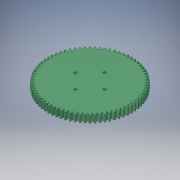
# Autodesk Inventor part: 000.302 - Втулка
Saved by Autodesk Inventor 2019 (Build 230136000, 136)
## iProperties
Created: 2020-02-27
Part Number: 000.302 - Втулка
Material: Пластик АБС
Document SubType Name: Modeling
Designer: Петров Иван
Density: 1.06 g/cm^3
Appearance: Гладкий — темный цвет морской волны
Author: Петров Иван
Autodesk Inventor part; units mm, degrees
ref_plane "YZ Plane" through (0, 0, 0) normal (1, 0, 0) x (0, 1, 0)
ref_plane "XZ Plane" through (0, 0, 0) normal (0, 1, 0) x (-1, 0, 0)
ref_plane "XY Plane" through (0, 0, 0) normal (0, 0, 1) x (1, 0, 0)
sketch "Эскиз1" plane through (0, 0, 0) normal (0, 1, 0) x (-1, 0, 0)
  circle A0 centre (0, 0) radius 12.5
  dimension "d0" = 25
  constraints: 1 centre point, 1 coincident
  measures "d0" diameter of A0
extrude "Выдавливание1" add sketch "Эскиз1" along normal blind 8
sketch "Эскиз2" plane through (0, 8, 0) normal (0, 1, 0) x (1, 0, 0)
  circle A0 centre (0, 0) radius 23
  dimension "d3" = 46
  constraints: 1 centre point, 1 coincident
  measures "d3" diameter of A0
extrude "Выдавливание2" add sketch "Эскиз2" along normal blind 2
sketch "Эскиз3" plane through (0, 10, 0) normal (0, 1, 0) x (1, 0, 0)
  arc A0 (-8.1938, 41.193) -> (-8.7829, 35.8928) centre (15.46, 35.881) ccw
  arc A1 (-8.7829, 35.8928) -> (-10.3402, 35.4755) centre (0, 0) ccw
  arc A2 (-10.3402, 35.4755) -> (-13.5005, 39.7711) centre (-31.3293, 23.3439) ccw
  arc A3 (-13.5005, 39.7711) -> (-15.2224, 39.1443) centre (0, 0) ccw
  arc A4 (-15.2224, 39.1443) -> (-14.8822, 33.8224) centre (8.9945, 38.0205) ccw
  arc A5 (-14.8822, 33.8224) -> (-16.3433, 33.141) centre (0, 0) ccw
  arc A6 (-16.3433, 33.141) -> (-20.2015, 36.8225) centre (-34.9069, 17.549) ccw
  arc A7 (-20.2015, 36.8225) -> (-21.7885, 35.9063) centre (0, 0) ccw
  arc A8 (-21.7885, 35.9063) -> (-20.5293, 30.7243) centre (2.2556, 39.0048) ccw
  arc A9 (-20.5293, 30.7243) -> (-21.8499, 29.7995) centre (0, 0) ccw
  arc A10 (-21.8499, 29.7995) -> (-26.2888, 32.7551) centre (-37.424, 11.2208) ccw
  arc A11 (-26.2888, 32.7551) -> (-27.6925, 31.5773) centre (0, 0) ccw
  arc A12 (-27.6925, 31.5773) -> (-25.5526, 26.6926) centre (-4.5518, 38.8039) ccw
  arc A13 (-25.5526, 26.6926) -> (-26.6926, 25.5526) centre (0, 0) ccw
  arc A14 (-26.6926, 25.5526) -> (-31.5773, 27.6925) centre (-38.8039, 4.5518) ccw
  arc A15 (-31.5773, 27.6925) -> (-32.7551, 26.2888) centre (0, 0) ccw
  arc A16 (-32.7551, 26.2888) -> (-29.7995, 21.8499) centre (-11.2208, 37.424) ccw
  arc A17 (-29.7995, 21.8499) -> (-30.7243, 20.5293) centre (0, 0) ccw
  arc A18 (-30.7243, 20.5293) -> (-35.9063, 21.7885) centre (-39.0048, -2.2556) ccw
  arc A19 (-35.9063, 21.7885) -> (-36.8225, 20.2015) centre (0, 0) ccw
  arc A20 (-36.8225, 20.2015) -> (-33.141, 16.3433) centre (-17.549, 34.9069) ccw
  arc A21 (-33.141, 16.3433) -> (-33.8224, 14.8822) centre (0, 0) ccw
  arc A22 (-33.8224, 14.8822) -> (-39.1443, 15.2224) centre (-38.0205, -8.9945) ccw
  arc A23 (-39.1443, 15.2224) -> (-39.7711, 13.5005) centre (0, 0) ccw
  arc A24 (-39.7711, 13.5005) -> (-35.4755, 10.3402) centre (-23.3439, 31.3293) ccw
  arc A25 (-35.4755, 10.3402) -> (-35.8928, 8.7829) centre (0, 0) ccw
  arc A26 (-35.8928, 8.7829) -> (-41.193, 8.1938) centre (-35.881, -15.46) ccw
  arc A27 (-41.193, 8.1938) -> (-41.5112, 6.3892) centre (0, 0) ccw
  arc A28 (-41.5112, 6.3892) -> (-36.7321, 4.0228) centre (-28.4295, 26.7997) ccw
  arc A29 (-36.7321, 4.0228) -> (-36.8726, 2.4168) centre (0, 0) ccw
  arc A30 (-36.8726, 2.4168) -> (-41.99, 0.9162) centre (-32.6513, -21.4558) ccw
  arc A31 (-41.99, 0.9162) -> (-41.99, -0.9162) centre (0, 0) ccw
  arc A32 (-41.99, -0.9162) -> (-36.8726, -2.4168) centre (-32.6513, 21.4558) ccw
  arc A33 (-36.8726, -2.4168) -> (-36.7321, -4.0228) centre (0, 0) ccw
  arc A34 (-36.7321, -4.0228) -> (-41.5112, -6.3892) centre (-28.4295, -26.7997) ccw
  arc A35 (-41.5112, -6.3892) -> (-41.193, -8.1938) centre (0, 0) ccw
  arc A36 (-41.193, -8.1938) -> (-35.8928, -8.7829) centre (-35.881, 15.46) ccw
  arc A37 (-35.8928, -8.7829) -> (-35.4755, -10.3402) centre (0, 0) ccw
  arc A38 (-35.4755, -10.3402) -> (-39.7711, -13.5005) centre (-23.3439, -31.3293) ccw
  arc A39 (-39.7711, -13.5005) -> (-39.1443, -15.2224) centre (0, 0) ccw
  arc A40 (-39.1443, -15.2224) -> (-33.8224, -14.8822) centre (-38.0205, 8.9945) ccw
  arc A41 (-33.8224, -14.8822) -> (-33.141, -16.3433) centre (0, 0) ccw
  arc A42 (-33.141, -16.3433) -> (-36.8225, -20.2015) centre (-17.549, -34.9069) ccw
  arc A43 (-36.8225, -20.2015) -> (-35.9063, -21.7885) centre (0, 0) ccw
  arc A44 (-35.9063, -21.7885) -> (-30.7243, -20.5293) centre (-39.0048, 2.2556) ccw
  arc A45 (-30.7243, -20.5293) -> (-29.7995, -21.8499) centre (0, 0) ccw
  arc A46 (-29.7995, -21.8499) -> (-32.7551, -26.2888) centre (-11.2208, -37.424) ccw
  arc A47 (-32.7551, -26.2888) -> (-31.5773, -27.6925) centre (0, 0) ccw
  arc A48 (-31.5773, -27.6925) -> (-26.6926, -25.5526) centre (-38.8039, -4.5518) ccw
  arc A49 (-26.6926, -25.5526) -> (-25.5526, -26.6926) centre (0, 0) ccw
  arc A50 (-25.5526, -26.6926) -> (-27.6925, -31.5773) centre (-4.5518, -38.8039) ccw
  arc A51 (-27.6925, -31.5773) -> (-26.2888, -32.7551) centre (0, 0) ccw
  arc A52 (-26.2888, -32.7551) -> (-21.8499, -29.7995) centre (-37.424, -11.2208) ccw
  arc A53 (-21.8499, -29.7995) -> (-20.5293, -30.7243) centre (0, 0) ccw
  arc A54 (-20.5293, -30.7243) -> (-21.7885, -35.9063) centre (2.2556, -39.0048) ccw
  arc A55 (-21.7885, -35.9063) -> (-20.2015, -36.8225) centre (0, 0) ccw
  arc A56 (-20.2015, -36.8225) -> (-16.3433, -33.141) centre (-34.9069, -17.549) ccw
  arc A57 (-16.3433, -33.141) -> (-14.8822, -33.8224) centre (0, 0) ccw
  arc A58 (-14.8822, -33.8224) -> (-15.2224, -39.1443) centre (8.9945, -38.0205) ccw
  arc A59 (-15.2224, -39.1443) -> (-13.5005, -39.7711) centre (0, 0) ccw
  arc A60 (-13.5005, -39.7711) -> (-10.3402, -35.4755) centre (-31.3293, -23.3439) ccw
  arc A61 (-10.3402, -35.4755) -> (-8.7829, -35.8928) centre (0, 0) ccw
  arc A62 (-8.7829, -35.8928) -> (-8.1938, -41.193) centre (15.46, -35.881) ccw
  arc A63 (-8.1938, -41.193) -> (-6.3892, -41.5112) centre (0, 0) ccw
  arc A64 (-6.3892, -41.5112) -> (-4.0228, -36.7321) centre (-26.7997, -28.4295) ccw
  arc A65 (-4.0228, -36.7321) -> (-2.4168, -36.8726) centre (0, 0) ccw
  arc A66 (-2.4168, -36.8726) -> (-0.9162, -41.99) centre (21.4558, -32.6513) ccw
  arc A67 (-0.9162, -41.99) -> (0.9162, -41.99) centre (0, 0) ccw
  arc A68 (0.9162, -41.99) -> (2.4168, -36.8726) centre (-21.4558, -32.6513) ccw
  arc A69 (2.4168, -36.8726) -> (4.0228, -36.7321) centre (0, 0) ccw
  arc A70 (4.0228, -36.7321) -> (6.3892, -41.5112) centre (26.7997, -28.4295) ccw
  arc A71 (6.3892, -41.5112) -> (8.1938, -41.193) centre (0, 0) ccw
  arc A72 (8.1938, -41.193) -> (8.7829, -35.8928) centre (-15.46, -35.881) ccw
  arc A73 (8.7829, -35.8928) -> (10.3402, -35.4755) centre (0, 0) ccw
  arc A74 (10.3402, -35.4755) -> (13.5005, -39.7711) centre (31.3293, -23.3439) ccw
  arc A75 (13.5005, -39.7711) -> (15.2224, -39.1443) centre (0, 0) ccw
  arc A76 (15.2224, -39.1443) -> (14.8822, -33.8224) centre (-8.9945, -38.0205) ccw
  arc A77 (14.8822, -33.8224) -> (16.3433, -33.141) centre (0, 0) ccw
  arc A78 (16.3433, -33.141) -> (20.2015, -36.8225) centre (34.9069, -17.549) ccw
  arc A79 (20.2015, -36.8225) -> (21.7885, -35.9063) centre (0, 0) ccw
  arc A80 (21.7885, -35.9063) -> (20.5293, -30.7243) centre (-2.2556, -39.0048) ccw
  arc A81 (20.5293, -30.7243) -> (21.8499, -29.7995) centre (0, 0) ccw
  arc A82 (21.8499, -29.7995) -> (26.2888, -32.7551) centre (37.424, -11.2208) ccw
  arc A83 (26.2888, -32.7551) -> (27.6925, -31.5773) centre (0, 0) ccw
  arc A84 (27.6925, -31.5773) -> (25.5526, -26.6926) centre (4.5518, -38.8039) ccw
  arc A85 (25.5526, -26.6926) -> (26.6926, -25.5526) centre (0, 0) ccw
  arc A86 (26.6926, -25.5526) -> (31.5773, -27.6925) centre (38.8039, -4.5518) ccw
  arc A87 (31.5773, -27.6925) -> (32.7551, -26.2888) centre (0, 0) ccw
  arc A88 (32.7551, -26.2888) -> (29.7995, -21.8499) centre (11.2208, -37.424) ccw
  arc A89 (29.7995, -21.8499) -> (30.7243, -20.5293) centre (0, 0) ccw
  arc A90 (30.7243, -20.5293) -> (35.9063, -21.7885) centre (39.0048, 2.2556) ccw
  arc A91 (35.9063, -21.7885) -> (36.8225, -20.2015) centre (0, 0) ccw
  arc A92 (36.8225, -20.2015) -> (33.141, -16.3433) centre (17.549, -34.9069) ccw
  arc A93 (33.141, -16.3433) -> (33.8224, -14.8822) centre (0, 0) ccw
  arc A94 (33.8224, -14.8822) -> (39.1443, -15.2224) centre (38.0205, 8.9945) ccw
  arc A95 (39.1443, -15.2224) -> (39.7711, -13.5005) centre (0, 0) ccw
  arc A96 (39.7711, -13.5005) -> (35.4755, -10.3402) centre (23.3439, -31.3293) ccw
  arc A97 (35.4755, -10.3402) -> (35.8928, -8.7829) centre (0, 0) ccw
  arc A98 (35.8928, -8.7829) -> (41.193, -8.1938) centre (35.881, 15.46) ccw
  arc A99 (41.193, -8.1938) -> (41.5112, -6.3892) centre (0, 0) ccw
  arc A100 (41.5112, -6.3892) -> (36.7321, -4.0228) centre (28.4295, -26.7997) ccw
  arc A101 (36.7321, -4.0228) -> (36.8726, -2.4168) centre (0, 0) ccw
  arc A102 (36.8726, -2.4168) -> (41.99, -0.9162) centre (32.6513, 21.4558) ccw
  arc A103 (41.99, -0.9162) -> (41.99, 0.9162) centre (0, 0) ccw
  arc A104 (41.99, 0.9162) -> (36.8726, 2.4168) centre (32.6513, -21.4558) ccw
  arc A105 (36.8726, 2.4168) -> (36.7321, 4.0228) centre (0, 0) ccw
  arc A106 (36.7321, 4.0228) -> (41.5112, 6.3892) centre (28.4295, 26.7997) ccw
  arc A107 (41.5112, 6.3892) -> (41.193, 8.1938) centre (0, 0) ccw
  arc A108 (41.193, 8.1938) -> (35.8928, 8.7829) centre (35.881, -15.46) ccw
  arc A109 (35.8928, 8.7829) -> (35.4755, 10.3402) centre (0, 0) ccw
  arc A110 (35.4755, 10.3402) -> (39.7711, 13.5005) centre (23.3439, 31.3293) ccw
  arc A111 (39.7711, 13.5005) -> (39.1443, 15.2224) centre (0, 0) ccw
  arc A112 (39.1443, 15.2224) -> (33.8224, 14.8822) centre (38.0205, -8.9945) ccw
  arc A113 (33.8224, 14.8822) -> (33.141, 16.3433) centre (0, 0) ccw
  arc A114 (33.141, 16.3433) -> (36.8225, 20.2015) centre (17.549, 34.9069) ccw
  arc A115 (36.8225, 20.2015) -> (35.9063, 21.7885) centre (0, 0) ccw
  arc A116 (35.9063, 21.7885) -> (30.7243, 20.5293) centre (39.0048, -2.2556) ccw
  arc A117 (30.7243, 20.5293) -> (29.7995, 21.8499) centre (0, 0) ccw
  arc A118 (29.7995, 21.8499) -> (32.7551, 26.2888) centre (11.2208, 37.424) ccw
  arc A119 (32.7551, 26.2888) -> (31.5773, 27.6925) centre (0, 0) ccw
  arc A120 (31.5773, 27.6925) -> (26.6926, 25.5526) centre (38.8039, 4.5518) ccw
  arc A121 (26.6926, 25.5526) -> (25.5526, 26.6926) centre (0, 0) ccw
  arc A122 (25.5526, 26.6926) -> (27.6925, 31.5773) centre (4.5518, 38.8039) ccw
  arc A123 (27.6925, 31.5773) -> (26.2888, 32.7551) centre (0, 0) ccw
  arc A124 (26.2888, 32.7551) -> (21.8499, 29.7995) centre (37.424, 11.2208) ccw
  arc A125 (21.8499, 29.7995) -> (20.5293, 30.7243) centre (0, 0) ccw
  arc A126 (20.5293, 30.7243) -> (21.7885, 35.9063) centre (-2.2556, 39.0048) ccw
  arc A127 (21.7885, 35.9063) -> (20.2015, 36.8225) centre (0, 0) ccw
  arc A128 (20.2015, 36.8225) -> (16.3433, 33.141) centre (34.9069, 17.549) ccw
  arc A129 (16.3433, 33.141) -> (14.8822, 33.8224) centre (0, 0) ccw
  arc A130 (14.8822, 33.8224) -> (15.2224, 39.1443) centre (-8.9945, 38.0205) ccw
  arc A131 (15.2224, 39.1443) -> (13.5005, 39.7711) centre (0, 0) ccw
  arc A132 (13.5005, 39.7711) -> (10.3402, 35.4755) centre (31.3293, 23.3439) ccw
  arc A133 (10.3402, 35.4755) -> (8.7829, 35.8928) centre (0, 0) ccw
  arc A134 (8.7829, 35.8928) -> (8.1938, 41.193) centre (-15.46, 35.881) ccw
  arc A135 (8.1938, 41.193) -> (6.3892, 41.5112) centre (0, 0) ccw
  arc A136 (6.3892, 41.5112) -> (4.0228, 36.7321) centre (26.7997, 28.4295) ccw
  arc A137 (4.0228, 36.7321) -> (2.4168, 36.8726) centre (0, 0) ccw
  arc A138 (2.4168, 36.8726) -> (0.9162, 41.99) centre (-21.4558, 32.6513) ccw
  arc A139 (0.9162, 41.99) -> (-0.9162, 41.99) centre (0, 0) ccw
  arc A140 (-0.9162, 41.99) -> (-2.4168, 36.8726) centre (21.4558, 32.6513) ccw
  arc A141 (-2.4168, 36.8726) -> (-4.0228, 36.7321) centre (0, 0) ccw
  arc A142 (-4.0228, 36.7321) -> (-6.3892, 41.5112) centre (-26.7997, 28.4295) ccw
  arc A143 (-6.3892, 41.5112) -> (-8.1938, 41.193) centre (0, 0) ccw
  arc A144 (4.8028, -48.7641) -> (5.506, -45.6664) centre (-12.0114, -43.3185) ccw
  arc A145 (5.506, -45.6664) -> (6.5009, -45.5354) centre (0, 0) ccw
  arc A146 (6.5009, -45.5354) -> (7.9819, -48.3455) centre (22.8137, -38.7337) ccw
  arc A147 (7.9819, -48.3455) -> (9.0346, -48.1599) centre (0, 0) ccw
  arc A148 (9.0346, -48.1599) -> (9.4652, -45.0127) centre (-8.1902, -44.2005) ccw
  arc A149 (9.4652, -45.0127) -> (10.4449, -44.7955) centre (0, 0) ccw
  arc A150 (10.4449, -44.7955) -> (12.1651, -47.4659) centre (26.1028, -36.598) ccw
  arc A151 (12.1651, -47.4659) -> (13.1977, -47.1892) centre (0, 0) ccw
  arc A152 (13.1977, -47.1892) -> (13.3523, -44.0165) centre (-4.3067, -44.7461) ccw
  arc A153 (13.3523, -44.0165) -> (14.3093, -43.7148) centre (0, 0) ccw
  arc A154 (14.3093, -43.7148) -> (16.2557, -46.225) centre (29.1932, -34.1837) ccw
  arc A155 (16.2557, -46.225) -> (17.2603, -45.8594) centre (0, 0) ccw
  arc A156 (17.2603, -45.8594) -> (17.1377, -42.6853) centre (-0.3904, -44.9512) ccw
  arc A157 (17.1377, -42.6853) -> (18.0648, -42.3013) centre (0, 0) ccw
  arc A158 (18.0648, -42.3013) -> (20.2226, -44.6323) centre (32.0614, -31.5092) ccw
  arc A159 (20.2226, -44.6323) -> (21.1915, -44.1806) centre (0, 0) ccw
  arc A160 (21.1915, -44.1806) -> (20.7928, -41.0292) centre (3.5288, -44.8142) ccw
  arc A161 (20.7928, -41.0292) -> (21.6829, -40.5658) centre (0, 0) ccw
  arc A162 (21.6829, -40.5658) -> (24.0357, -42.7) centre (34.6856, -28.595) ccw
  arc A163 (24.0357, -42.7) -> (24.9614, -42.1655) centre (0, 0) ccw
  arc A164 (24.9614, -42.1655) -> (24.2896, -39.0609) centre (7.4212, -44.3361) ccw
  arc A165 (24.2896, -39.0609) -> (25.1359, -38.5217) centre (0, 0) ccw
  arc A166 (25.1359, -38.5217) -> (27.6657, -40.4426) centre (37.0458, -25.4632) ccw
  arc A167 (27.6657, -40.4426) -> (28.5414, -39.8295) centre (0, 0) ccw
  arc A168 (28.5414, -39.8295) -> (27.6016, -36.7952) centre (11.2571, -43.5206) ccw
  arc A169 (27.6016, -36.7952) -> (28.3977, -36.1844) centre (0, 0) ccw
  arc A170 (28.3977, -36.1844) -> (31.0853, -37.8775) centre (39.1241, -22.1375) ccw
  arc A171 (31.0853, -37.8775) -> (31.9042, -37.1904) centre (0, 0) ccw
  arc A172 (31.9042, -37.1904) -> (30.7034, -34.2496) centre (15.0073, -42.3739) ccw
  arc A173 (30.7034, -34.2496) -> (31.4433, -33.5717) centre (0, 0) ccw
  arc A174 (31.4433, -33.5717) -> (34.2682, -35.0241) centre (40.9046, -18.6434) ccw
  arc A175 (34.2682, -35.0241) -> (35.0241, -34.2682) centre (0, 0) ccw
  arc A176 (35.0241, -34.2682) -> (33.5717, -31.4433) centre (18.6434, -40.9046) ccw
  arc A177 (33.5717, -31.4433) -> (34.2496, -30.7034) centre (0, 0) ccw
  arc A178 (34.2496, -30.7034) -> (37.1904, -31.9042) centre (42.3739, -15.0073) ccw
  arc A179 (37.1904, -31.9042) -> (37.8775, -31.0853) centre (0, 0) ccw
  arc A180 (37.8775, -31.0853) -> (36.1844, -28.3977) centre (22.1375, -39.1241) ccw
  arc A181 (36.1844, -28.3977) -> (36.7952, -27.6016) centre (0, 0) ccw
  arc A182 (36.7952, -27.6016) -> (39.8295, -28.5414) centre (43.5206, -11.2571) ccw
  arc A183 (39.8295, -28.5414) -> (40.4426, -27.6657) centre (0, 0) ccw
  arc A184 (40.4426, -27.6657) -> (38.5217, -25.1359) centre (25.4632, -37.0458) ccw
  arc A185 (38.5217, -25.1359) -> (39.0609, -24.2896) centre (0, 0) ccw
  arc A186 (39.0609, -24.2896) -> (42.1655, -24.9614) centre (44.3361, -7.4212) ccw
  arc A187 (42.1655, -24.9614) -> (42.7, -24.0357) centre (0, 0) ccw
  arc A188 (42.7, -24.0357) -> (40.5658, -21.6829) centre (28.595, -34.6856) ccw
  arc A189 (40.5658, -21.6829) -> (41.0292, -20.7928) centre (0, 0) ccw
  arc A190 (41.0292, -20.7928) -> (44.1806, -21.1915) centre (44.8142, -3.5288) ccw
  arc A191 (44.1806, -21.1915) -> (44.6323, -20.2226) centre (0, 0) ccw
  arc A192 (44.6323, -20.2226) -> (42.3013, -18.0648) centre (31.5092, -32.0614) ccw
  arc A193 (42.3013, -18.0648) -> (42.6853, -17.1377) centre (0, 0) ccw
  arc A194 (42.6853, -17.1377) -> (45.8594, -17.2603) centre (44.9512, 0.3904) ccw
  arc A195 (45.8594, -17.2603) -> (46.225, -16.2557) centre (0, 0) ccw
  arc A196 (46.225, -16.2557) -> (43.7148, -14.3093) centre (34.1837, -29.1932) ccw
  arc A197 (43.7148, -14.3093) -> (44.0165, -13.3523) centre (0, 0) ccw
  arc A198 (44.0165, -13.3523) -> (47.1892, -13.1977) centre (44.7461, 4.3067) ccw
  arc A199 (47.1892, -13.1977) -> (47.4659, -12.1651) centre (0, 0) ccw
  arc A200 (47.4659, -12.1651) -> (44.7955, -10.4449) centre (36.598, -26.1028) ccw
  arc A201 (44.7955, -10.4449) -> (45.0127, -9.4652) centre (0, 0) ccw
  arc A202 (45.0127, -9.4652) -> (48.1599, -9.0346) centre (44.2005, 8.1902) ccw
  arc A203 (48.1599, -9.0346) -> (48.3455, -7.9819) centre (0, 0) ccw
  arc A204 (48.3455, -7.9819) -> (45.5354, -6.5009) centre (38.7337, -22.8137) ccw
  arc A205 (45.5354, -6.5009) -> (45.6664, -5.506) centre (0, 0) ccw
  arc A206 (45.6664, -5.506) -> (48.7641, -4.8028) centre (43.3185, 12.0114) ccw
  arc A207 (48.7641, -4.8028) -> (48.8572, -3.7379) centre (0, 0) ccw
  arc A208 (48.8572, -3.7379) -> (45.9287, -2.5075) centre (40.5746, -19.3511) ccw
  arc A209 (45.9287, -2.5075) -> (45.9725, -1.505) centre (0, 0) ccw
  arc A210 (45.9725, -1.505) -> (48.9971, -0.5345) centre (42.1068, 15.7411) ccw
  arc A211 (48.9971, -0.5345) -> (48.9971, 0.5345) centre (0, 0) ccw
  arc A212 (48.9971, 0.5345) -> (45.9725, 1.505) centre (42.1068, -15.7411) ccw
  arc A213 (45.9725, 1.505) -> (45.9287, 2.5075) centre (0, 0) ccw
  arc A214 (45.9287, 2.5075) -> (48.8572, 3.7379) centre (40.5746, 19.3511) ccw
  arc A215 (48.8572, 3.7379) -> (48.7641, 4.8028) centre (0, 0) ccw
  arc A216 (48.7641, 4.8028) -> (45.6664, 5.506) centre (43.3185, -12.0114) ccw
  arc A217 (45.6664, 5.506) -> (45.5354, 6.5009) centre (0, 0) ccw
  arc A218 (45.5354, 6.5009) -> (48.3455, 7.9819) centre (38.7337, 22.8137) ccw
  arc A219 (48.3455, 7.9819) -> (48.1599, 9.0346) centre (0, 0) ccw
  arc A220 (48.1599, 9.0346) -> (45.0127, 9.4652) centre (44.2005, -8.1902) ccw
  arc A221 (45.0127, 9.4652) -> (44.7955, 10.4449) centre (0, 0) ccw
  arc A222 (44.7955, 10.4449) -> (47.4659, 12.1651) centre (36.598, 26.1028) ccw
  arc A223 (47.4659, 12.1651) -> (47.1892, 13.1977) centre (0, 0) ccw
  arc A224 (47.1892, 13.1977) -> (44.0165, 13.3523) centre (44.7461, -4.3067) ccw
  arc A225 (44.0165, 13.3523) -> (43.7148, 14.3093) centre (0, 0) ccw
  arc A226 (43.7148, 14.3093) -> (46.225, 16.2557) centre (34.1837, 29.1932) ccw
  arc A227 (46.225, 16.2557) -> (45.8594, 17.2603) centre (0, 0) ccw
  arc A228 (45.8594, 17.2603) -> (42.6853, 17.1377) centre (44.9512, -0.3904) ccw
  arc A229 (42.6853, 17.1377) -> (42.3013, 18.0648) centre (0, 0) ccw
  arc A230 (42.3013, 18.0648) -> (44.6323, 20.2226) centre (31.5092, 32.0614) ccw
  arc A231 (44.6323, 20.2226) -> (44.1806, 21.1915) centre (0, 0) ccw
  arc A232 (44.1806, 21.1915) -> (41.0292, 20.7928) centre (44.8142, 3.5288) ccw
  arc A233 (41.0292, 20.7928) -> (40.5658, 21.6829) centre (0, 0) ccw
  arc A234 (40.5658, 21.6829) -> (42.7, 24.0357) centre (28.595, 34.6856) ccw
  arc A235 (42.7, 24.0357) -> (42.1655, 24.9614) centre (0, 0) ccw
  arc A236 (42.1655, 24.9614) -> (39.0609, 24.2896) centre (44.3361, 7.4212) ccw
  arc A237 (39.0609, 24.2896) -> (38.5217, 25.1359) centre (0, 0) ccw
  arc A238 (38.5217, 25.1359) -> (40.4426, 27.6657) centre (25.4632, 37.0458) ccw
  arc A239 (40.4426, 27.6657) -> (39.8295, 28.5414) centre (0, 0) ccw
  arc A240 (39.8295, 28.5414) -> (36.7952, 27.6016) centre (43.5206, 11.2571) ccw
  arc A241 (36.7952, 27.6016) -> (36.1844, 28.3977) centre (0, 0) ccw
  arc A242 (36.1844, 28.3977) -> (37.8775, 31.0853) centre (22.1375, 39.1241) ccw
  arc A243 (37.8775, 31.0853) -> (37.1904, 31.9042) centre (0, 0) ccw
  arc A244 (37.1904, 31.9042) -> (34.2496, 30.7034) centre (42.3739, 15.0073) ccw
  arc A245 (34.2496, 30.7034) -> (33.5717, 31.4433) centre (0, 0) ccw
  arc A246 (33.5717, 31.4433) -> (35.0241, 34.2682) centre (18.6434, 40.9046) ccw
  arc A247 (35.0241, 34.2682) -> (34.2682, 35.0241) centre (0, 0) ccw
  arc A248 (34.2682, 35.0241) -> (31.4433, 33.5717) centre (40.9046, 18.6434) ccw
  arc A249 (31.4433, 33.5717) -> (30.7034, 34.2496) centre (0, 0) ccw
  arc A250 (30.7034, 34.2496) -> (31.9042, 37.1904) centre (15.0073, 42.3739) ccw
  arc A251 (31.9042, 37.1904) -> (31.0853, 37.8775) centre (0, 0) ccw
  arc A252 (31.0853, 37.8775) -> (28.3977, 36.1844) centre (39.1241, 22.1375) ccw
  arc A253 (28.3977, 36.1844) -> (27.6016, 36.7952) centre (0, 0) ccw
  arc A254 (27.6016, 36.7952) -> (28.5414, 39.8295) centre (11.2571, 43.5206) ccw
  arc A255 (28.5414, 39.8295) -> (27.6657, 40.4426) centre (0, 0) ccw
  arc A256 (27.6657, 40.4426) -> (25.1359, 38.5217) centre (37.0458, 25.4632) ccw
  arc A257 (25.1359, 38.5217) -> (24.2896, 39.0609) centre (0, 0) ccw
  arc A258 (24.2896, 39.0609) -> (24.9614, 42.1655) centre (7.4212, 44.3361) ccw
  arc A259 (24.9614, 42.1655) -> (24.0357, 42.7) centre (0, 0) ccw
  arc A260 (24.0357, 42.7) -> (21.6829, 40.5658) centre (34.6856, 28.595) ccw
  arc A261 (21.6829, 40.5658) -> (20.7928, 41.0292) centre (0, 0) ccw
  arc A262 (20.7928, 41.0292) -> (21.1915, 44.1806) centre (3.5288, 44.8142) ccw
  arc A263 (21.1915, 44.1806) -> (20.2226, 44.6323) centre (0, 0) ccw
  arc A264 (20.2226, 44.6323) -> (18.0648, 42.3013) centre (32.0614, 31.5092) ccw
  arc A265 (18.0648, 42.3013) -> (17.1377, 42.6853) centre (0, 0) ccw
  arc A266 (17.1377, 42.6853) -> (17.2603, 45.8594) centre (-0.3904, 44.9512) ccw
  arc A267 (17.2603, 45.8594) -> (16.2557, 46.225) centre (0, 0) ccw
  arc A268 (16.2557, 46.225) -> (14.3093, 43.7148) centre (29.1932, 34.1837) ccw
  arc A269 (14.3093, 43.7148) -> (13.3523, 44.0165) centre (0, 0) ccw
  arc A270 (13.3523, 44.0165) -> (13.1977, 47.1892) centre (-4.3067, 44.7461) ccw
  arc A271 (13.1977, 47.1892) -> (12.1651, 47.4659) centre (0, 0) ccw
  arc A272 (12.1651, 47.4659) -> (10.4449, 44.7955) centre (26.1028, 36.598) ccw
  arc A273 (10.4449, 44.7955) -> (9.4652, 45.0127) centre (0, 0) ccw
  arc A274 (9.4652, 45.0127) -> (9.0346, 48.1599) centre (-8.1902, 44.2005) ccw
  arc A275 (9.0346, 48.1599) -> (7.9819, 48.3455) centre (0, 0) ccw
  arc A276 (7.9819, 48.3455) -> (6.5009, 45.5354) centre (22.8137, 38.7337) ccw
  arc A277 (6.5009, 45.5354) -> (5.506, 45.6664) centre (0, 0) ccw
  arc A278 (5.506, 45.6664) -> (4.8028, 48.7641) centre (-12.0114, 43.3185) ccw
  arc A279 (4.8028, 48.7641) -> (3.7379, 48.8572) centre (0, 0) ccw
  arc A280 (3.7379, 48.8572) -> (2.5075, 45.9287) centre (19.3511, 40.5746) ccw
  arc A281 (2.5075, 45.9287) -> (1.505, 45.9725) centre (0, 0) ccw
  arc A282 (1.505, 45.9725) -> (0.5345, 48.9971) centre (-15.7411, 42.1068) ccw
  arc A283 (0.5345, 48.9971) -> (-0.5345, 48.9971) centre (0, 0) ccw
  arc A284 (-0.5345, 48.9971) -> (-1.505, 45.9725) centre (15.7411, 42.1068) ccw
  arc A285 (-1.505, 45.9725) -> (-2.5075, 45.9287) centre (0, 0) ccw
  arc A286 (-2.5075, 45.9287) -> (-3.7379, 48.8572) centre (-19.3511, 40.5746) ccw
  arc A287 (3.7379, -48.8572) -> (4.8028, -48.7641) centre (0, 0) ccw
  arc A288 (-4.8028, 48.7641) -> (-5.506, 45.6664) centre (12.0114, 43.3185) ccw
  arc A289 (-5.506, 45.6664) -> (-6.5009, 45.5354) centre (0, 0) ccw
  arc A290 (-6.5009, 45.5354) -> (-7.9819, 48.3455) centre (-22.8137, 38.7337) ccw
  arc A291 (-7.9819, 48.3455) -> (-9.0346, 48.1599) centre (0, 0) ccw
  arc A292 (-9.0346, 48.1599) -> (-9.4652, 45.0127) centre (8.1902, 44.2005) ccw
  arc A293 (-9.4652, 45.0127) -> (-10.4449, 44.7955) centre (0, 0) ccw
  arc A294 (-10.4449, 44.7955) -> (-12.1651, 47.4659) centre (-26.1028, 36.598) ccw
  arc A295 (-12.1651, 47.4659) -> (-13.1977, 47.1892) centre (0, 0) ccw
  arc A296 (-13.1977, 47.1892) -> (-13.3523, 44.0165) centre (4.3067, 44.7461) ccw
  arc A297 (-13.3523, 44.0165) -> (-14.3093, 43.7148) centre (0, 0) ccw
  arc A298 (-14.3093, 43.7148) -> (-16.2557, 46.225) centre (-29.1932, 34.1837) ccw
  arc A299 (-16.2557, 46.225) -> (-17.2603, 45.8594) centre (0, 0) ccw
  arc A300 (-17.2603, 45.8594) -> (-17.1377, 42.6853) centre (0.3904, 44.9512) ccw
  arc A301 (-17.1377, 42.6853) -> (-18.0648, 42.3013) centre (0, 0) ccw
  arc A302 (-18.0648, 42.3013) -> (-20.2226, 44.6323) centre (-32.0614, 31.5092) ccw
  arc A303 (-20.2226, 44.6323) -> (-21.1915, 44.1806) centre (0, 0) ccw
  arc A304 (-21.1915, 44.1806) -> (-20.7928, 41.0292) centre (-3.5288, 44.8142) ccw
  arc A305 (-20.7928, 41.0292) -> (-21.6829, 40.5658) centre (0, 0) ccw
  arc A306 (-21.6829, 40.5658) -> (-24.0357, 42.7) centre (-34.6856, 28.595) ccw
  arc A307 (-24.0357, 42.7) -> (-24.9614, 42.1655) centre (0, 0) ccw
  arc A308 (-24.9614, 42.1655) -> (-24.2896, 39.0609) centre (-7.4212, 44.3361) ccw
  arc A309 (-24.2896, 39.0609) -> (-25.1359, 38.5217) centre (0, 0) ccw
  arc A310 (-25.1359, 38.5217) -> (-27.6657, 40.4426) centre (-37.0458, 25.4632) ccw
  arc A311 (-27.6657, 40.4426) -> (-28.5414, 39.8295) centre (0, 0) ccw
  arc A312 (-28.5414, 39.8295) -> (-27.6016, 36.7952) centre (-11.2571, 43.5206) ccw
  arc A313 (-27.6016, 36.7952) -> (-28.3977, 36.1844) centre (0, 0) ccw
  arc A314 (-28.3977, 36.1844) -> (-31.0853, 37.8775) centre (-39.1241, 22.1375) ccw
  arc A315 (-31.0853, 37.8775) -> (-31.9042, 37.1904) centre (0, 0) ccw
  arc A316 (-31.9042, 37.1904) -> (-30.7034, 34.2496) centre (-15.0073, 42.3739) ccw
  arc A317 (-30.7034, 34.2496) -> (-31.4433, 33.5717) centre (0, 0) ccw
  arc A318 (-31.4433, 33.5717) -> (-34.2682, 35.0241) centre (-40.9046, 18.6434) ccw
  arc A319 (-34.2682, 35.0241) -> (-35.0241, 34.2682) centre (0, 0) ccw
  arc A320 (-35.0241, 34.2682) -> (-33.5717, 31.4433) centre (-18.6434, 40.9046) ccw
  arc A321 (-33.5717, 31.4433) -> (-34.2496, 30.7034) centre (0, 0) ccw
  arc A322 (-34.2496, 30.7034) -> (-37.1904, 31.9042) centre (-42.3739, 15.0073) ccw
  arc A323 (-37.1904, 31.9042) -> (-37.8775, 31.0853) centre (0, 0) ccw
  arc A324 (-37.8775, 31.0853) -> (-36.1844, 28.3977) centre (-22.1375, 39.1241) ccw
  arc A325 (-36.1844, 28.3977) -> (-36.7952, 27.6016) centre (0, 0) ccw
  arc A326 (-36.7952, 27.6016) -> (-39.8295, 28.5414) centre (-43.5206, 11.2571) ccw
  arc A327 (-39.8295, 28.5414) -> (-40.4426, 27.6657) centre (0, 0) ccw
  arc A328 (-40.4426, 27.6657) -> (-38.5217, 25.1359) centre (-25.4632, 37.0458) ccw
  arc A329 (-38.5217, 25.1359) -> (-39.0609, 24.2896) centre (0, 0) ccw
  arc A330 (-39.0609, 24.2896) -> (-42.1655, 24.9614) centre (-44.3361, 7.4212) ccw
  arc A331 (-42.1655, 24.9614) -> (-42.7, 24.0357) centre (0, 0) ccw
  arc A332 (-42.7, 24.0357) -> (-40.5658, 21.6829) centre (-28.595, 34.6856) ccw
  arc A333 (-40.5658, 21.6829) -> (-41.0292, 20.7928) centre (0, 0) ccw
  arc A334 (-41.0292, 20.7928) -> (-44.1806, 21.1915) centre (-44.8142, 3.5288) ccw
  arc A335 (-44.1806, 21.1915) -> (-44.6323, 20.2226) centre (0, 0) ccw
  arc A336 (-44.6323, 20.2226) -> (-42.3013, 18.0648) centre (-31.5092, 32.0614) ccw
  arc A337 (-42.3013, 18.0648) -> (-42.6853, 17.1377) centre (0, 0) ccw
  arc A338 (-42.6853, 17.1377) -> (-45.8594, 17.2603) centre (-44.9512, -0.3904) ccw
  arc A339 (-45.8594, 17.2603) -> (-46.225, 16.2557) centre (0, 0) ccw
  arc A340 (-46.225, 16.2557) -> (-43.7148, 14.3093) centre (-34.1837, 29.1932) ccw
  arc A341 (-43.7148, 14.3093) -> (-44.0165, 13.3523) centre (0, 0) ccw
  arc A342 (-44.0165, 13.3523) -> (-47.1892, 13.1977) centre (-44.7461, -4.3067) ccw
  arc A343 (-47.1892, 13.1977) -> (-47.4659, 12.1651) centre (0, 0) ccw
  arc A344 (-47.4659, 12.1651) -> (-44.7955, 10.4449) centre (-36.598, 26.1028) ccw
  arc A345 (-44.7955, 10.4449) -> (-45.0127, 9.4652) centre (0, 0) ccw
  arc A346 (-45.0127, 9.4652) -> (-48.1599, 9.0346) centre (-44.2005, -8.1902) ccw
  arc A347 (-48.1599, 9.0346) -> (-48.3455, 7.9819) centre (0, 0) ccw
  arc A348 (-48.3455, 7.9819) -> (-45.5354, 6.5009) centre (-38.7337, 22.8137) ccw
  arc A349 (-45.5354, 6.5009) -> (-45.6664, 5.506) centre (0, 0) ccw
  arc A350 (-45.6664, 5.506) -> (-48.7641, 4.8028) centre (-43.3185, -12.0114) ccw
  arc A351 (-48.7641, 4.8028) -> (-48.8572, 3.7379) centre (0, 0) ccw
  arc A352 (-48.8572, 3.7379) -> (-45.9287, 2.5075) centre (-40.5746, 19.3511) ccw
  arc A353 (-45.9287, 2.5075) -> (-45.9725, 1.505) centre (0, 0) ccw
  arc A354 (-45.9725, 1.505) -> (-48.9971, 0.5345) centre (-42.1068, -15.7411) ccw
  arc A355 (-48.9971, 0.5345) -> (-48.9971, -0.5345) centre (0, 0) ccw
  arc A356 (-48.9971, -0.5345) -> (-45.9725, -1.505) centre (-42.1068, 15.7411) ccw
  arc A357 (-45.9725, -1.505) -> (-45.9287, -2.5075) centre (0, 0) ccw
  arc A358 (-45.9287, -2.5075) -> (-48.8572, -3.7379) centre (-40.5746, -19.3511) ccw
  arc A359 (-48.8572, -3.7379) -> (-48.7641, -4.8028) centre (0, 0) ccw
  arc A360 (-48.7641, -4.8028) -> (-45.6664, -5.506) centre (-43.3185, 12.0114) ccw
  arc A361 (-45.6664, -5.506) -> (-45.5354, -6.5009) centre (0, 0) ccw
  arc A362 (-45.5354, -6.5009) -> (-48.3455, -7.9819) centre (-38.7337, -22.8137) ccw
  arc A363 (-48.3455, -7.9819) -> (-48.1599, -9.0346) centre (0, 0) ccw
  arc A364 (-48.1599, -9.0346) -> (-45.0127, -9.4652) centre (-44.2005, 8.1902) ccw
  arc A365 (-45.0127, -9.4652) -> (-44.7955, -10.4449) centre (0, 0) ccw
  arc A366 (-44.7955, -10.4449) -> (-47.4659, -12.1651) centre (-36.598, -26.1028) ccw
  arc A367 (-47.4659, -12.1651) -> (-47.1892, -13.1977) centre (0, 0) ccw
  arc A368 (-47.1892, -13.1977) -> (-44.0165, -13.3523) centre (-44.7461, 4.3067) ccw
  arc A369 (-44.0165, -13.3523) -> (-43.7148, -14.3093) centre (0, 0) ccw
  arc A370 (-43.7148, -14.3093) -> (-46.225, -16.2557) centre (-34.1837, -29.1932) ccw
  arc A371 (-46.225, -16.2557) -> (-45.8594, -17.2603) centre (0, 0) ccw
  arc A372 (-45.8594, -17.2603) -> (-42.6853, -17.1377) centre (-44.9512, 0.3904) ccw
  arc A373 (-42.6853, -17.1377) -> (-42.3013, -18.0648) centre (0, 0) ccw
  arc A374 (-42.3013, -18.0648) -> (-44.6323, -20.2226) centre (-31.5092, -32.0614) ccw
  arc A375 (-44.6323, -20.2226) -> (-44.1806, -21.1915) centre (0, 0) ccw
  arc A376 (-44.1806, -21.1915) -> (-41.0292, -20.7928) centre (-44.8142, -3.5288) ccw
  arc A377 (-41.0292, -20.7928) -> (-40.5658, -21.6829) centre (0, 0) ccw
  arc A378 (-40.5658, -21.6829) -> (-42.7, -24.0357) centre (-28.595, -34.6856) ccw
  arc A379 (-42.7, -24.0357) -> (-42.1655, -24.9614) centre (0, 0) ccw
  arc A380 (-42.1655, -24.9614) -> (-39.0609, -24.2896) centre (-44.3361, -7.4212) ccw
  arc A381 (-39.0609, -24.2896) -> (-38.5217, -25.1359) centre (0, 0) ccw
  arc A382 (-38.5217, -25.1359) -> (-40.4426, -27.6657) centre (-25.4632, -37.0458) ccw
  arc A383 (-40.4426, -27.6657) -> (-39.8295, -28.5414) centre (0, 0) ccw
  arc A384 (-39.8295, -28.5414) -> (-36.7952, -27.6016) centre (-43.5206, -11.2571) ccw
  arc A385 (-36.7952, -27.6016) -> (-36.1844, -28.3977) centre (0, 0) ccw
  arc A386 (-36.1844, -28.3977) -> (-37.8775, -31.0853) centre (-22.1375, -39.1241) ccw
  arc A387 (-37.8775, -31.0853) -> (-37.1904, -31.9042) centre (0, 0) ccw
  arc A388 (-37.1904, -31.9042) -> (-34.2496, -30.7034) centre (-42.3739, -15.0073) ccw
  arc A389 (-34.2496, -30.7034) -> (-33.5717, -31.4433) centre (0, 0) ccw
  arc A390 (-33.5717, -31.4433) -> (-35.0241, -34.2682) centre (-18.6434, -40.9046) ccw
  arc A391 (-35.0241, -34.2682) -> (-34.2682, -35.0241) centre (0, 0) ccw
  arc A392 (-34.2682, -35.0241) -> (-31.4433, -33.5717) centre (-40.9046, -18.6434) ccw
  arc A393 (-31.4433, -33.5717) -> (-30.7034, -34.2496) centre (0, 0) ccw
  arc A394 (-30.7034, -34.2496) -> (-31.9042, -37.1904) centre (-15.0073, -42.3739) ccw
  arc A395 (-31.9042, -37.1904) -> (-31.0853, -37.8775) centre (0, 0) ccw
  arc A396 (-31.0853, -37.8775) -> (-28.3977, -36.1844) centre (-39.1241, -22.1375) ccw
  arc A397 (-28.3977, -36.1844) -> (-27.6016, -36.7952) centre (0, 0) ccw
  arc A398 (-27.6016, -36.7952) -> (-28.5414, -39.8295) centre (-11.2571, -43.5206) ccw
  arc A399 (-28.5414, -39.8295) -> (-27.6657, -40.4426) centre (0, 0) ccw
  arc A400 (-27.6657, -40.4426) -> (-25.1359, -38.5217) centre (-37.0458, -25.4632) ccw
  arc A401 (-25.1359, -38.5217) -> (-24.2896, -39.0609) centre (0, 0) ccw
  arc A402 (-24.2896, -39.0609) -> (-24.9614, -42.1655) centre (-7.4212, -44.3361) ccw
  arc A403 (-24.9614, -42.1655) -> (-24.0357, -42.7) centre (0, 0) ccw
  arc A404 (-24.0357, -42.7) -> (-21.6829, -40.5658) centre (-34.6856, -28.595) ccw
  arc A405 (-21.6829, -40.5658) -> (-20.7928, -41.0292) centre (0, 0) ccw
  arc A406 (-20.7928, -41.0292) -> (-21.1915, -44.1806) centre (-3.5288, -44.8142) ccw
  arc A407 (-21.1915, -44.1806) -> (-20.2226, -44.6323) centre (0, 0) ccw
  arc A408 (-20.2226, -44.6323) -> (-18.0648, -42.3013) centre (-32.0614, -31.5092) ccw
  arc A409 (-18.0648, -42.3013) -> (-17.1377, -42.6853) centre (0, 0) ccw
  arc A410 (-17.1377, -42.6853) -> (-17.2603, -45.8594) centre (0.3904, -44.9512) ccw
  arc A411 (-17.2603, -45.8594) -> (-16.2557, -46.225) centre (0, 0) ccw
  arc A412 (-16.2557, -46.225) -> (-14.3093, -43.7148) centre (-29.1932, -34.1837) ccw
  arc A413 (-14.3093, -43.7148) -> (-13.3523, -44.0165) centre (0, 0) ccw
  arc A414 (-13.3523, -44.0165) -> (-13.1977, -47.1892) centre (4.3067, -44.7461) ccw
  arc A415 (-13.1977, -47.1892) -> (-12.1651, -47.4659) centre (0, 0) ccw
  arc A416 (-12.1651, -47.4659) -> (-10.4449, -44.7955) centre (-26.1028, -36.598) ccw
  arc A417 (-10.4449, -44.7955) -> (-9.4652, -45.0127) centre (0, 0) ccw
  arc A418 (-9.4652, -45.0127) -> (-9.0346, -48.1599) centre (8.1902, -44.2005) ccw
  arc A419 (-9.0346, -48.1599) -> (-7.9819, -48.3455) centre (0, 0) ccw
  arc A420 (-7.9819, -48.3455) -> (-6.5009, -45.5354) centre (-22.8137, -38.7337) ccw
  arc A421 (-6.5009, -45.5354) -> (-5.506, -45.6664) centre (0, 0) ccw
  arc A422 (-5.506, -45.6664) -> (-4.8028, -48.7641) centre (12.0114, -43.3185) ccw
  arc A423 (-4.8028, -48.7641) -> (-3.7379, -48.8572) centre (0, 0) ccw
  arc A424 (-3.7379, -48.8572) -> (-2.5075, -45.9287) centre (-19.3511, -40.5746) ccw
  arc A425 (-2.5075, -45.9287) -> (-1.505, -45.9725) centre (0, 0) ccw
  arc A426 (-1.505, -45.9725) -> (-0.5345, -48.9971) centre (15.7411, -42.1068) ccw
  arc A427 (-0.5345, -48.9971) -> (0.5345, -48.9971) centre (0, 0) ccw
  arc A428 (0.5345, -48.9971) -> (1.505, -45.9725) centre (-15.7411, -42.1068) ccw
  arc A429 (1.505, -45.9725) -> (2.5075, -45.9287) centre (0, 0) ccw
  arc A430 (2.5075, -45.9287) -> (3.7379, -48.8572) centre (19.3511, -40.5746) ccw
  arc A431 (-3.7379, 48.8572) -> (-4.8028, 48.7641) centre (0, 0) ccw
  constraints: 864 point on circle, 432 centre point
extrude "Выдавливание3" add sketch "Эскиз3" along normal blind 8 contours A143 A142 A141 A140 A139 A138 A137 A136 A135 A134 A133 A132 A131 A130 A129 A128 A127 A126 A125 A124 A123 A122 A121 A120 A119 A118 A117 A116 A115 A114 A113 A112 A111 A110 A109 A108 A107 A106 A105 A104 A103 A102 A101 A100 A99 A98 A97 A96 A95 A94 A93 A92 A91 A90 A89 A88 A87 A86 A85 A84 A83 A82 A81 A80 A79 A78 A77 A76 A75 A74 A73 A72 A71 A70 A69 A68 A67 A66 A65 A64 A63 A62 A61 A60 A59 A58 A57 A56 A55 A54 A53 A52 A51 A50 A49 A48 A47 A46 A45 A44 A43 A42 A41 A40 A39 A38 A37 A36 A35 A34 A33 A32 A31 A30 A29 A28 A27 A26 A25 A24 A23 A22 A21 A20 A19 A18 A17 A16 A15 A14 A13 A12 A11 A10 A9 A8 A7 A6 A5 A4 A3 A2 A1 A0 | A287 A430 A429 A428 A427 A426 A425 A424 A423 A422 A421 A420 A419 A418 A417 A416 A415 A414 A413 A412 A411 A410 A409 A408 A407 A406 A405 A404 A403 A402 A401 A400 A399 A398 A397 A396 A395 A394 A393 A392 A391 A390 A389 A388 A387 A386 A385 A384 A383 A382 A381 A380 A379 A378 A377 A376 A375 A374 A373 A372 A371 A370 A369 A368 A367 A366 A365 A364 A363 A362 A361 A360 A359 A358 A357 A356 A355 A354 A353 A352 A351 A350 A349 A348 A347 A346 A345 A344 A343 A342 A341 A340 A339 A338 A337 A336 A335 A334 A333 A332 A331 A330 A329 A328 A327 A326 A325 A324 A323 A322 A321 A320 A319 A318 A317 A316 A315 A314 A313 A312 A311 A310 A309 A308 A307 A306 A305 A304 A303 A302 A301 A300 A299 A298 A297 A296 A295 A294 A293 A292 A291 A290 A289 A288 A431 A286 A285 A284 A283 A282 A281 A280 A279 A278 A277 A276 A275 A274 A273 A272 A271 A270 A269 A268 A267 A266 A265 A264 A263 A262 A261 A260 A259 A258 A257 A256 A255 A254 A253 A252 A251 A250 A249 A248 A247 A246 A245 A244 A243 A242 A241 A240 A239 A238 A237 A236 A235 A234 A233 A232 A231 A230 A229 A228 A227 A226 A225 A224 A223 A222 A221 A220 A219 A218 A217 A216 A215 A214 A213 A212 A211 A210 A209 A208 A207 A206 A205 A204 A203 A202 A201 A200 A199 A198 A197 A196 A195 A194 A193 A192 A191 A190 A189 A188 A187 A186 A185 A184 A183 A182 A181 A180 A179 A178 A177 A176 A175 A174 A173 A172 A171 A170 A169 A168 A167 A166 A165 A164 A163 A162 A161 A160 A159 A158 A157 A156 A155 A154 A153 A152 A151 A150 A149 A148 A147 A146 A145 A144
sketch "Эскиз4" plane through (0, 8, 0) normal (0, -1, 0) x (1, 0, 0)
  line L0 (0, 0) -> (0, -17)
  line L1 (4, -17) -> (2, -20.4641)
  line L2 (2, -20.4641) -> (-2, -20.4641)
  line L3 (-2, -20.4641) -> (-4, -17)
  line L4 (-4, -17) -> (-2, -13.5359)
  line L5 (-2, -13.5359) -> (2, -13.5359)
  line L6 (2, -13.5359) -> (4, -17)
  dimension "d8" = 17
  dimension "d9" = 8
  constraints: 14 end point, 1 coincident, 1 vertical, 13 other
  measures "d8" distance of L0.start L0.end
  measures "d9" distance of L3.end L1.start
extrude "Выдавливание4" cut sketch "Эскиз4" against normal blind 3.3
sketch "Эскиз6" plane through (0, 11.3, 0) normal (0, -1, 0) x (1, 0, 0)
  circle A0 centre (0, 0) radius 12.5 projected
  line L0 (0, 0) -> (0, -17)
  line L1 (3.05, -17) -> (1.525, -19.6414)
  line L2 (1.525, -19.6414) -> (-1.525, -19.6414)
  line L3 (-1.525, -19.6414) -> (-3.05, -17)
  line L4 (-3.05, -17) -> (-1.525, -14.3586)
  line L5 (-1.525, -14.3586) -> (1.525, -14.3586)
  line L6 (1.525, -14.3586) -> (3.05, -17)
  dimension "d16" = 17
  dimension "d17" = 6.1
  constraints: 14 end point, 1 coincident, 1 vertical, 13 other
  measures "d16" distance of L0.start L0.end
  measures "d17" distance of L3.end L1.start
extrude "Выдавливание6" cut sketch "Эскиз6" against normal blind 2.6 contours L5 L6 L1 L2 L3 L4
sketch "Эскиз7" plane through (0, 13.9, 0) normal (0, -1, 0) x (1, 0, 0)
  circle A0 centre (0, 0) radius 12.5 projected
  line L0 (0, 0) -> (0, -17)
  circle A1 centre (0, -17) radius 1.5
  dimension "d20" = 17
  dimension "d21" = 3
  constraints: 2 end point, 1 centre point, 1 coincident, 1 vertical
  measures "d20" distance of L0.start L0.end
  measures "d21" diameter of A1
extrude "Выдавливание7" cut sketch "Эскиз7" against normal through all contours A1
pattern_circular "Круговой массив1" count 4 over 360 about axis through (0, 0, 0) along (0, 1, 0) of "Выдавливание6", "Выдавливание7", "Выдавливание4"
sketch "Эскиз8" plane through (0, 0, 0) normal (0, -1, 0) x (1, 0, 0)
  circle A0 centre (0, 0) radius 5.375
  circle A1 centre (0, 0) radius 3.375
  line L0 (-6.9327, -1) -> (-6.9327, 1)
  line L1 (-6.9327, 1) -> (-6.9327, 1.5)
  line L2 (-8.2327, 1.5) -> (-6.9327, 1.5)
  spline S0 degree 3 poles (-8.308, 1) (-8.3, 1.0653) (-8.2914, 1.1299) (-8.274, 1.2508) (-8.2654, 1.3061) (-8.2506, 1.3973) (-8.2444, 1.4332) (-8.2376, 1.4723) (-8.2358, 1.4829) (-8.2345, 1.49) (-8.2345, 1.4901) (-8.2345, 1.4902) (-8.2339, 1.4935) (-8.2333, 1.4967) (-8.2327, 1.5) knots -0.079145 -0.079145 -0.079145 -0.079145 -0.059419 -0.059419 -0.039575 -0.039575 -0.020572 -0.020572 -0.010101 -0.010101 -0.009923 -0.009923 -0.009923 -0.004948 -0.004948 -0.004948 -0.004948
  ellipse E0 centre (-0.8138, 2.2378) end of major axis (-6.2384, -4.8493) minor radius 6.6293 (-8.308, 1) -> (-8.3138, -1) ccw
  line L3 (-6.9327, -1.5) -> (-8.2327, -1.5)
  line L4 (-6.9327, -1.5) -> (-6.9327, -1)
  spline S1 degree 3 poles (-8.2327, -1.5) (-8.2334, -1.4968) (-8.234, -1.4935) (-8.2347, -1.4903) (-8.2347, -1.4901) (-8.2347, -1.49) (-8.2361, -1.4829) (-8.2382, -1.4724) (-8.2457, -1.4333) (-8.2525, -1.3974) (-8.2687, -1.3062) (-8.278, -1.2509) (-8.2965, -1.1299) (-8.3056, -1.0653) (-8.3138, -1) knots -0.074295 -0.074295 -0.074295 -0.074295 -0.069327 -0.069327 -0.069327 -0.069138 -0.069138 -0.058667 -0.058667 -0.039648 -0.039648 -0.019752 -0.019752 -0.000001 -0.000001 -0.000001 -0.000001
  line L5 (2.8341, 0.75) -> (-2.8341, 0.75)
  line L6 (2.8929, 0.7945) -> (2.8341, 0.75)
  arc A2 (2.8929, 0.7945) -> (2.8468, 0.9465) centre (0, 0) ccw
  line L7 (2.3559, 0.9758) -> (2.8468, 0.9465)
  line L8 (2.6823, 1.3437) -> (2.3559, 0.9758)
  arc A3 (2.6823, 1.3437) -> (2.6074, 1.4837) centre (0, 0) ccw
  line L9 (2.1202, 1.4167) -> (2.6074, 1.4837)
  line L10 (2.3686, 1.8411) -> (2.1202, 1.4167)
  arc A4 (2.3686, 1.8411) -> (2.2678, 1.9639) centre (0, 0) ccw
  line L11 (1.8031, 1.8031) -> (2.2678, 1.9639)
  line L12 (1.9639, 2.2678) -> (1.8031, 1.8031)
  arc A5 (1.9639, 2.2678) -> (1.8411, 2.3686) centre (0, 0) ccw
  line L13 (1.4167, 2.1202) -> (1.8411, 2.3686)
  line L14 (1.4837, 2.6074) -> (1.4167, 2.1202)
  arc A6 (1.4837, 2.6074) -> (1.3437, 2.6823) centre (0, 0) ccw
  line L15 (0.9758, 2.3559) -> (1.3437, 2.6823)
  line L16 (0.9465, 2.8468) -> (0.9758, 2.3559)
  arc A7 (0.9465, 2.8468) -> (0.7945, 2.8929) centre (0, 0) ccw
  line L17 (0.4975, 2.501) -> (0.7945, 2.8929)
  line L18 (0.373, 2.9767) -> (0.4975, 2.501)
  arc A8 (0.373, 2.9767) -> (0.2149, 2.9923) centre (0, 0) ccw
  line L19 (0, 2.55) -> (0.2149, 2.9923)
  line L20 (-0.2149, 2.9923) -> (0, 2.55)
  arc A9 (-0.2149, 2.9923) -> (-0.373, 2.9767) centre (0, 0) ccw
  line L21 (-0.4975, 2.501) -> (-0.373, 2.9767)
  line L22 (-0.7945, 2.8929) -> (-0.4975, 2.501)
  arc A10 (-0.7945, 2.8929) -> (-0.9465, 2.8468) centre (0, 0) ccw
  line L23 (-0.9758, 2.3559) -> (-0.9465, 2.8468)
  line L24 (-1.3437, 2.6823) -> (-0.9758, 2.3559)
  arc A11 (-1.3437, 2.6823) -> (-1.4837, 2.6074) centre (0, 0) ccw
  line L25 (-1.4167, 2.1202) -> (-1.4837, 2.6074)
  line L26 (-1.8411, 2.3686) -> (-1.4167, 2.1202)
  arc A12 (-1.8411, 2.3686) -> (-1.9639, 2.2678) centre (0, 0) ccw
  line L27 (-1.8031, 1.8031) -> (-1.9639, 2.2678)
  line L28 (-2.2678, 1.9639) -> (-1.8031, 1.8031)
  arc A13 (-2.2678, 1.9639) -> (-2.3686, 1.8411) centre (0, 0) ccw
  line L29 (-2.1202, 1.4167) -> (-2.3686, 1.8411)
  line L30 (-2.6074, 1.4837) -> (-2.1202, 1.4167)
  arc A14 (-2.6074, 1.4837) -> (-2.6823, 1.3437) centre (0, 0) ccw
  line L31 (-2.3559, 0.9758) -> (-2.6823, 1.3437)
  line L32 (-2.8468, 0.9465) -> (-2.3559, 0.9758)
  arc A15 (-2.8468, 0.9465) -> (-2.8929, 0.7945) centre (0, 0) ccw
  line L33 (-2.8341, 0.75) -> (-2.8929, 0.7945)
  arc A16 (-2.8929, 0.7945) -> (-2.8929, -0.7945) centre (0, 0) ccw
  line L34 (2.8929, 0.7945) -> (2.8341, 0.75)
  line L35 (2.8341, 0.75) -> (-2.8341, 0.75)
  line L36 (-2.8341, 0.75) -> (-2.8929, 0.7945)
  arc A17 (-2.8929, 0.7945) -> (-2.8929, -0.7945) centre (0, 0) ccw
  line L37 (-2.8929, -0.7945) -> (-2.8341, -0.75)
  line L38 (-2.8341, -0.75) -> (2.8341, -0.75)
  line L39 (2.8341, -0.75) -> (2.8929, -0.7945)
  arc A18 (2.8929, -0.7945) -> (2.8929, 0.7945) centre (0, 0) ccw
  line L40 (-2.8341, -0.75) -> (2.8341, -0.75)
  line L41 (-2.8929, -0.7945) -> (-2.8341, -0.75)
  arc A19 (-2.8929, -0.7945) -> (-2.8468, -0.9465) centre (0, 0) ccw
  line L42 (-2.3559, -0.9758) -> (-2.8468, -0.9465)
  line L43 (-2.6823, -1.3437) -> (-2.3559, -0.9758)
  arc A20 (-2.6823, -1.3437) -> (-2.6074, -1.4837) centre (0, 0) ccw
  line L44 (-2.1202, -1.4167) -> (-2.6074, -1.4837)
  line L45 (-2.3686, -1.8411) -> (-2.1202, -1.4167)
  arc A21 (-2.3686, -1.8411) -> (-2.2678, -1.9639) centre (0, 0) ccw
  line L46 (-1.8031, -1.8031) -> (-2.2678, -1.9639)
  line L47 (-1.9639, -2.2678) -> (-1.8031, -1.8031)
  arc A22 (-1.9639, -2.2678) -> (-1.8411, -2.3686) centre (0, 0) ccw
  line L48 (-1.4167, -2.1202) -> (-1.8411, -2.3686)
  line L49 (-1.4837, -2.6074) -> (-1.4167, -2.1202)
  arc A23 (-1.4837, -2.6074) -> (-1.3437, -2.6823) centre (0, 0) ccw
  line L50 (-0.9758, -2.3559) -> (-1.3437, -2.6823)
  line L51 (-0.9465, -2.8468) -> (-0.9758, -2.3559)
  arc A24 (-0.9465, -2.8468) -> (-0.7945, -2.8929) centre (0, 0) ccw
  line L52 (-0.4975, -2.501) -> (-0.7945, -2.8929)
  line L53 (-0.373, -2.9767) -> (-0.4975, -2.501)
  arc A25 (-0.373, -2.9767) -> (-0.2149, -2.9923) centre (0, 0) ccw
  line L54 (0, -2.55) -> (-0.2149, -2.9923)
  line L55 (0.2149, -2.9923) -> (0, -2.55)
  arc A26 (0.2149, -2.9923) -> (0.373, -2.9767) centre (0, 0) ccw
  line L56 (0.4975, -2.501) -> (0.373, -2.9767)
  line L57 (0.7945, -2.8929) -> (0.4975, -2.501)
  arc A27 (0.7945, -2.8929) -> (0.9465, -2.8468) centre (0, 0) ccw
  line L58 (0.9758, -2.3559) -> (0.9465, -2.8468)
  line L59 (1.3437, -2.6823) -> (0.9758, -2.3559)
  arc A28 (1.3437, -2.6823) -> (1.4837, -2.6074) centre (0, 0) ccw
  line L60 (1.4167, -2.1202) -> (1.4837, -2.6074)
  line L61 (1.8411, -2.3686) -> (1.4167, -2.1202)
  arc A29 (1.8411, -2.3686) -> (1.9639, -2.2678) centre (0, 0) ccw
  line L62 (1.8031, -1.8031) -> (1.9639, -2.2678)
  line L63 (2.2678, -1.9639) -> (1.8031, -1.8031)
  arc A30 (2.2678, -1.9639) -> (2.3686, -1.8411) centre (0, 0) ccw
  line L64 (2.1202, -1.4167) -> (2.3686, -1.8411)
  line L65 (2.6074, -1.4837) -> (2.1202, -1.4167)
  arc A31 (2.6074, -1.4837) -> (2.6823, -1.3437) centre (0, 0) ccw
  line L66 (2.3559, -0.9758) -> (2.6823, -1.3437)
  line L67 (2.8468, -0.9465) -> (2.3559, -0.9758)
  arc A32 (2.8468, -0.9465) -> (2.8929, -0.7945) centre (0, 0) ccw
  line L68 (2.8341, -0.75) -> (2.8929, -0.7945)
  constraints: 138 end point, 62 point on circle, 33 centre point, 8 other
extrude "Выдавливание8" cut sketch "Эскиз8" against normal blind 10 contours L5 L33 A15 L32 L31 A14 L30 L29 A13 L28 L27 A12 L26 L25 A11 L24 L23 A10 L22 L21 A9 L20 L19 A8 L18 L17 A7 L16 L15 A6 L14 L13 A5 L12 L11 A4 L10 L9 A3 L8 L7 A2 L6 | A32 L67 L66 A31 L65 L64 A30 L63 L62 A29 L61 L60 A28 L59 L58 A27 L57 L56 A26 L55 L54 A25 L53 L52 A24 L51 L50 A23 L49 L48 A22 L47 L46 A21 L45 L44 A20 L43 L42 A19 L37 L38 L39
